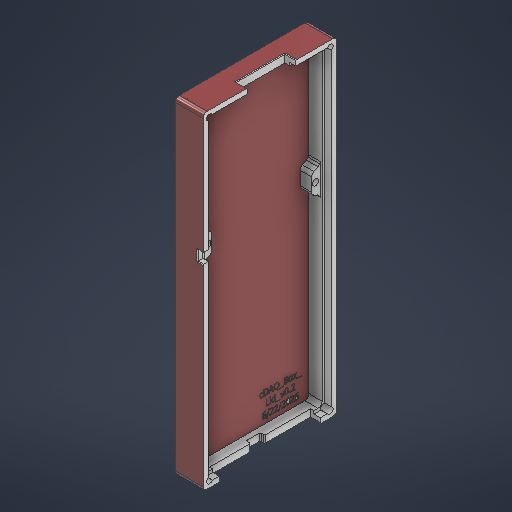
# Autodesk Inventor part: cDAQ_Box_Lid_v0.2
Saved by Autodesk Inventor 2027 (Build 310192000, 192)
## iProperties
Created: 2026-05-08
Part Number: cDAQ_Box_Lid_v0.2
Material: Generic
Document SubType Name: Modeling
Designer: giese
Density: 1 g/cm^3
Appearance: Default
Author: giese
Autodesk Inventor part; units mm, degrees
(part 1 of 2)
ref_plane "YZ Plane" through (0, 0, 0) normal (1, 0, 0) x (0, 1, 0)
ref_plane "XZ Plane" through (0, 0, 0) normal (0, 1, 0) x (-1, 0, 0)
ref_plane "XY Plane" through (0, 0, 0) normal (0, 0, 1) x (1, 0, 0)
sketch "Sketch1" plane through (0, 0, 0) normal (1, 0, 0) x (0, 1, 0)
  line L0 (50.7569, 48.4212) -> (-204.2591, 48.4212)
  line L1 (-204.2591, 48.4212) -> (-204.2591, -55.7188)
  line L2 (-204.2591, -55.7188) -> (50.7569, -55.7188)
  line L3 (50.7569, -55.7188) -> (50.7569, 48.4212)
  point P0 (0, 0)
  dimension "d0" = 104.14
  dimension "d1" = 255.016
  constraints: 8 end point, 2 parallel, 1 horizontal, 1 perpendicular
  measures "d0" distance of L2.end L0.start
  measures "d1" distance of L0.start L0.end
extrude "Extrusion1" add sketch "Sketch1" along normal blind 21.59
sketch "Sketch2" plane through (21.59, 0, 0) normal (1, 0, 0) x (0, 0, -1)
  line L0 (-42.0712, 44.4069) -> (49.3688, 44.4069)
  line L1 (49.3688, 44.4069) -> (49.3688, -197.9091)
  line L2 (49.3688, -197.9091) -> (-42.0712, -197.9091)
  line L3 (-42.0712, -197.9091) -> (-42.0712, 44.4069)
  line L4 (-48.4212, 50.7569) -> (-48.4212, -204.2591) projected
  line L5 (-48.4212, -204.2591) -> (55.7188, -204.2591) projected
  point P0 (0, 0)
  dimension "d4" = 91.44
  dimension "d5" = 242.316
  dimension "d6" = 6.35
  dimension "d7" = 6.35
  constraints: 8 end point, 2 parallel, 1 horizontal, 1 perpendicular
  measures "d4" distance of L0.start L0.end
  measures "d5" distance of L0.end L1.end
  measures "d6" distance between parallel lines of L4 L3
  measures "d7" distance between parallel lines of L5 L2
extrude "Extrusion2" cut sketch "Sketch2" against normal blind 15.24
sketch "Sketch3" plane through (0, 0, 0) normal (-1, 0, 0) x (0, 0, 1)
  circle A0 centre (-32.8588, 7.3229) radius 2
  line L0 (-55.7188, -204.2591) -> (-55.7188, 50.7569) projected
  line L1 (-55.7188, 50.7569) -> (48.4212, 50.7569) projected
  circle A1 centre (-14.36, 7.3229) radius 2
  circle A2 centre (4.1389, 7.3229) radius 2
  point P0 (0, 0)
  dimension "d10" = 22.86
  dimension "d11" = 43.434
  dimension "d12" = 43.434
  dimension "d13" = 18.4988
  dimension "d14" = 4
  dimension "d15" = 4
  dimension "d16" = 43.434
  dimension "d17" = 18.4988
  dimension "d18" = 36.9976
  dimension "d21" = 4
  constraints: 3 centre point
  measures "d10" distance from line of L0 A0.centre
  measures "d11" distance from line of L1 A0.centre
  measures "d12" distance from line of L1 A1.centre
  measures "d13" distance of A0.centre A1.centre
  measures "d14" diameter of A1
  measures "d15" diameter of A2
  measures "d16" distance from line of L1 A2.centre
  measures "d17" distance of A1.centre A2.centre
  measures "d18" distance of A0.centre A2.centre
  measures "d21" diameter of A0
extrude "Extrusion3" [suppressed]
sketch "Sketch6" plane through (0, 50.7569, 48.4212) normal (0, 1, 0) x (1, 0, 0)
  line L0 (21.59, 6.35) -> (21.59, 97.79) projected
  line L1 (12.954, 34.29) -> (21.59, 34.29)
  line L2 (21.59, 34.29) -> (21.59, 72.39)
  line L3 (21.59, 72.39) -> (12.954, 72.39)
  line L4 (12.954, 72.39) -> (12.954, 34.29)
  line L5 (0, 104.14) -> (21.59, 104.14) projected
  point P0 (0, 48.4212)
  point P1 (17.272, 72.39)
  point P2 (17.272, 34.29)
  dimension "d30" = 8.636
  dimension "d31" = 38.1
  dimension "d32" = 31.75
  constraints: 8 end point, 2 midpoint, 2 parallel, 1 horizontal, 1 perpendicular, 1 point on line
  measures "d30" distance between parallel lines of L0 L4
  measures "d31" distance of point (17.272, 72.39) point (17.272, 34.29)
  measures "d32" distance between parallel lines of L5 L3
extrude "Extrusion5" cut sketch "Sketch6" against normal blind 6.35
fillet "Fillet1" radius 3.175 4 edges at (10.795, 50.7569, -55.7188) (10.795, 50.7569, 48.4212) (10.795, -204.2591, 48.4212) (10.795, -204.2591, -55.7188)
sketch "Sketch7" plane through (21.59, 0, 0) normal (1, 0, 0) x (0, 0, -1)
  line L0 (-42.0712, -197.9091) -> (-42.0712, 44.4069) projected
  line L1 (-42.0712, 44.4069) -> (-42.3252, 44.4069)
  line L2 (-42.3252, 46.6929) -> (-44.2302, 46.6929)
  line L3 (-44.2302, 46.6929) -> (-44.2302, 51.0109)
  line L4 (-42.0712, -190.1621) -> (-42.0712, -197.9091)
  line L5 (49.3688, -197.9091) -> (-42.0712, -197.9091) projected
  line L6 (-40.4202, -200.1951) -> (-44.2302, -200.1951)
  line L7 (-44.2302, -200.1951) -> (-44.2302, -190.1621)
  line L8 (49.3688, 44.4069) -> (49.3688, -197.9091) projected
  line L9 (49.3688, -192.7021) -> (49.3688, -197.9091)
  line L10 (49.3688, -197.9091) -> (43.9078, -197.9091)
  line L11 (49.3688, -197.9091) -> (49.3688, -192.7021)
  line L12 (51.5278, -192.7021) -> (51.5278, -200.1951)
  line L13 (51.5278, -200.1951) -> (43.9078, -200.1951)
  line L14 (-42.0712, 44.4069) -> (49.3688, 44.4069) projected
  line L15 (42.0028, 44.4069) -> (49.3688, 44.4069)
  line L16 (51.5278, 48.4709) -> (51.5278, 46.6929)
  line L17 (51.5278, 46.6929) -> (42.0028, 46.6929)
  line L18 (-42.3252, 46.6929) -> (42.0028, 46.6929)
  line L19 (42.0028, 44.4069) -> (-42.3252, 44.4069)
  line L20 (51.5278, 48.4709) -> (51.5278, -192.7021)
  line L21 (44.2888, -195.2421) -> (44.2888, 44.4069)
  line L22 (43.9078, -197.9091) -> (-40.4202, -197.9091)
  line L23 (-40.4202, -200.1951) -> (43.9078, -200.1951)
  line L24 (-44.2302, -190.1621) -> (-44.2302, 51.0109)
  line L25 (-42.0712, 44.4069) -> (-42.0712, -190.1621)
  point P0 (0, 0)
  point P1 (-42.0712, 51.0109)
  point P2 (-44.2302, 48.9789)
  point P3 (49.3688, 48.4709)
  point P4 (51.5278, 46.6929)
  point P5 (-44.2302, 46.6929)
  point P6 (-42.0712, 50.7569)
  point P7 (46.8288, 50.7569)
  dimension "d34" = 2.286
  dimension "d35" = 2.159
  dimension "d38" = 2.159
  dimension "d39" = 2.286
  dimension "d42" = 2.286
  dimension "d43" = 2.159
  dimension "d46" = 2.286
  dimension "d47" = 2.159
  constraints: 44 end point, 7 point on line, 4 parallel, 4 perpendicular, 2 collinear, 2 horizontal, 2 vertical, 3 other
  measures "d34" distance between parallel lines of L2 L1
  measures "d35" distance between parallel lines of L0 L3
  measures "d38" distance between parallel lines of L7 L0
  measures "d39" distance between parallel lines of L5 L6
  measures "d42" distance between parallel lines of L5 L13
  measures "d46" distance between parallel lines of L14 L17
extrude "Extrusion6" cut sketch "Sketch7" against normal blind 5 contours L0 L14 L8 L5 | L18 L17 L20 L12 L13 L23 L6 L7 L24 L2
fillet "Fillet2" radius 3.175 8 edges at (19.09, 46.6929, 44.2302) (11.47, 44.4069, 42.0712) (19.09, 46.6929, -51.5278) (11.47, 44.4069, -49.3688) (11.47, -197.9091, 42.0712) (19.09, -200.1951, 44.2302) (11.47, -197.9091, -49.3688) (19.09, -200.1951, -51.5278)
sketch "Sketch11" plane through (16.59, 0, 0) normal (1, 0, 0) x (0, 0, -1)
  circle A0 centre (50.6388, 45.6769) radius 2.4005
  line L0 (52.5438, 50.7569) -> (23.9688, 50.7569) projected
  line L1 (55.7188, -201.0841) -> (55.7188, 47.5819) projected
  arc A1 (46.9238, 45.7719) -> (43.7488, 48.9469) centre (43.7488, 45.7719) ccw projected
  circle A2 centre (-43.3412, 45.6769) radius 2.4005
  line L2 (-48.4212, 47.5819) -> (-48.4212, -201.0841) projected
  line L3 (-14.1312, 50.7569) -> (-45.2462, 50.7569) projected
  circle A3 centre (50.6388, -199.1791) radius 2.4005
  line L4 (-45.2462, -204.2591) -> (52.5438, -204.2591) projected
  circle A4 centre (-43.3412, -199.1791) radius 2.4005
  circle A5 centre (45.5588, -45.7631) radius 2.4005
  circle A6 centre (-38.2612, -45.7631) radius 2.4005
  point P0 (0, 0)
  point P1 (45.9939, 48.017)
  point P2 (48.5528, -43.2993)
  point P3 (45.3778, -46.4743)
  point P4 (-30.4007, -42.8803)
  point P5 (-33.5757, -46.0553)
  point P6 (46.8288, 50.7569)
  point P7 (-42.0712, 50.7569)
  dimension "d58" = 4.801
  dimension "d59" = 5.08
  dimension "d60" = 5.08
  dimension "d61" = 4.801
  dimension "d62" = 4.801
  dimension "d63" = 5.08
  dimension "d64" = 5.08
  dimension "d65" = 4.801
  dimension "d66" = 5.08
  dimension "d67" = 5.08
  dimension "d76" = 5.08
  dimension "d77" = 5.08
  dimension "d114" = 4.801
  dimension "d115" = 96.52
  dimension "d116" = 10.16
  dimension "d117" = 4.801
  dimension "d118" = 96.52
  dimension "d119" = 10.16
  constraints: 6 centre point, 1 point on circle
  measures "d58" diameter of A0
  measures "d59" distance from line of L2 A2.centre
  measures "d60" distance from line of L3 A2.centre
  measures "d61" diameter of A2
  measures "d62" diameter of A3
  measures "d63" distance from line of L1 A3.centre
  measures "d64" distance from line of L4 A3.centre
  measures "d65" diameter of A4
  measures "d66" distance from line of L2 A4.centre
  measures "d67" distance from line of L4 A4.centre
  measures "d76" distance from line of L1 A0.centre
  measures "d77" distance from line of L0 A0.centre
  measures "d114" diameter of A5
  measures "d115" distance from line of A5.centre L0
  measures "d116" distance from line of L1 A5.centre
  measures "d117" diameter of A6
  measures "d118" distance from line of A6.centre L3
  measures "d119" distance from line of L2 A6.centre
extrude "Extrusion8" cut sketch "Sketch11" along normal blind 5.08 and the other way blind 17.78
sketch "Sketch13" plane through (6.35, 0, 0) normal (1, 0, 0) x (0, 0, -1)
  line L0 (14.7094, -174.4803) -> (39.7652, -174.4803) construction
  line L1 (39.7652, -174.4803) -> (39.7652, -183.3446) construction
  line L2 (39.7652, -183.3446) -> (14.7094, -183.3446) construction
  line L3 (14.7094, -183.3446) -> (14.7094, -174.4803) construction
  spline S0 degree 2 poles (12.7321, -179.2264) (12.3764, -179.2264) (11.7873, -179.0078) (11.5762, -178.7855) knots 0 0 0 1 2 2 2
  spline S1 degree 2 poles (11.5762, -178.7855) (11.365, -178.567) (11.1316, -177.8926) (11.1316, -177.4406) knots 0 0 0 1 2 2 2
  spline S2 degree 2 poles (11.1316, -177.4406) (11.1316, -176.9886) (11.3724, -176.3291) (11.5762, -176.1068) knots 0 0 0 1 2 2 2
  spline S3 degree 2 poles (11.5762, -176.1068) (11.7799, -175.8808) (12.3839, -175.64) (12.7321, -175.64) knots 0 0 0 1 2 2 2
  spline S4 degree 2 poles (12.7321, -175.64) (13.0137, -175.64) (13.5398, -175.7993) (13.7436, -175.903) knots 0 0 0 1 2 2 2
  line L4 (13.7436, -175.903) -> (13.7436, -176.5514)
  line L5 (13.7436, -176.5514) -> (13.7103, -176.5514)
  spline S5 degree 2 poles (13.7103, -176.5514) (13.6473, -176.4995) (13.4546, -176.3662) (13.3175, -176.2958) knots 0 0 0 1 2 2 2
  spline S6 degree 2 poles (13.3175, -176.2958) (13.1953, -176.2365) (12.8692, -176.1439) (12.721, -176.1439) knots 0 0 0 1 2 2 2
  spline S7 degree 2 poles (12.721, -176.1439) (12.2727, -176.1439) (11.7281, -176.8219) (11.7281, -177.4406) knots 0 0 0 1 2 2 2
  spline S8 degree 2 poles (11.7281, -177.4406) (11.7281, -178.0445) (12.2542, -178.7226) (12.721, -178.7226) knots 0 0 0 1 2 2 2
  spline S9 degree 2 poles (12.721, -178.7226) (13.0026, -178.7226) (13.5139, -178.4891) (13.7103, -178.3076) knots 0 0 0 1 2 2 2
  line L6 (13.7103, -178.3076) -> (13.7436, -178.3076)
  line L7 (13.7436, -178.3076) -> (13.7436, -178.956)
  spline S10 degree 2 poles (13.7436, -178.956) (13.6584, -178.9967) (13.399, -179.1116) (13.2953, -179.1375) knots 0 0 0 1 2 2 2
  spline S11 degree 2 poles (13.2953, -179.1375) (13.1471, -179.182) (12.9137, -179.2264) (12.7321, -179.2264) knots 0 0 0 1 2 2 2
  spline S12 degree 2 poles (17.9192, -176.8663) (17.9192, -177.4925) (17.4116, -178.5003) (16.9855, -178.7818) knots 0 0 0 1 2 2 2
  spline S13 degree 2 poles (16.9855, -178.7818) (16.6372, -179.0004) (15.9222, -179.1486) (15.3664, -179.1486) knots 0 0 0 1 2 2 2
  line L8 (15.3664, -179.1486) -> (14.3142, -179.1486)
  line L9 (14.3142, -179.1486) -> (14.3142, -174.5766)
  line L10 (14.3142, -174.5766) -> (15.3553, -174.5766)
  spline S14 degree 2 poles (15.3553, -174.5766) (16, -174.5766) (16.7336, -174.7693) (16.9929, -174.9397) knots 0 0 0 1 2 2 2
  spline S15 degree 2 poles (16.9929, -174.9397) (17.4338, -175.2324) (17.9192, -176.1994) (17.9192, -176.8663) knots 0 0 0 1 2 2 2
  spline S16 degree 2 poles (17.2856, -176.8589) (17.2856, -176.3328) (16.9373, -175.5881) (16.5928, -175.3769) knots 0 0 0 1 2 2 2
  spline S17 degree 2 poles (16.5928, -175.3769) (16.3482, -175.2324) (15.7962, -175.1028) (15.3849, -175.1028) knots 0 0 0 1 2 2 2
  line L11 (15.3849, -175.1028) -> (14.9218, -175.1028)
  line L12 (14.9218, -175.1028) -> (14.9218, -178.6225)
  line L13 (14.9218, -178.6225) -> (15.3849, -178.6225)
  spline S18 degree 2 poles (15.3849, -178.6225) (15.7888, -178.6225) (16.4001, -178.4929) (16.6483, -178.3187) knots 0 0 0 1 2 2 2
  spline S19 degree 2 poles (16.6483, -178.3187) (16.967, -178.1038) (17.2856, -177.3925) (17.2856, -176.8589) knots 0 0 0 1 2 2 2
  line L14 (18.0859, -179.1486) -> (19.6272, -174.5766)
  line L15 (19.6272, -174.5766) -> (20.3756, -174.5766)
  line L16 (20.3756, -174.5766) -> (21.9169, -179.1486)
  line L17 (21.9169, -179.1486) -> (21.2759, -179.1486)
  line L18 (21.2759, -179.1486) -> (20.8609, -177.8704)
  line L19 (20.8609, -177.8704) -> (19.1159, -177.8704)
  line L20 (19.1159, -177.8704) -> (18.7009, -179.1486)
  line L21 (18.7009, -179.1486) -> (18.0859, -179.1486)
  line L22 (20.6942, -177.3517) -> (19.9866, -175.1991)
  line L23 (19.9866, -175.1991) -> (19.2826, -177.3517)
  line L24 (19.2826, -177.3517) -> (20.6942, -177.3517)
  spline S20 degree 2 poles (26.148, -180.2676) (25.9813, -180.3083) (25.6182, -180.3528) (25.4367, -180.3528) knots 0 0 0 1 2 2 2
  spline S21 degree 2 poles (25.4367, -180.3528) (24.9217, -180.3528) (24.2807, -179.7785) (24.251, -179.245) knots 0 0 0 1 2 2 2
  spline S22 degree 2 poles (24.251, -179.245) (24.2103, -179.245) (24.1399, -179.245) (24.1103, -179.245) knots 0 0 0 1 2 2 2
  spline S23 degree 2 poles (24.1103, -179.245) (23.6471, -179.245) (22.9024, -178.93) (22.6357, -178.6225) knots 0 0 0 1 2 2 2
  spline S24 degree 2 poles (22.6357, -178.6225) (22.3726, -178.3187) (22.091, -177.4295) (22.091, -176.8663) knots 0 0 0 1 2 2 2
  spline S25 degree 2 poles (22.091, -176.8663) (22.091, -176.2884) (22.3763, -175.414) (22.6394, -175.1028) knots 0 0 0 1 2 2 2
  spline S26 degree 2 poles (22.6394, -175.1028) (22.9061, -174.7952) (23.6508, -174.4803) (24.1103, -174.4803) knots 0 0 0 1 2 2 2
  spline S27 degree 2 poles (24.1103, -174.4803) (24.5771, -174.4803) (25.3255, -174.8064) (25.5849, -175.1028) knots 0 0 0 1 2 2 2
  spline S28 degree 2 poles (25.5849, -175.1028) (25.8442, -175.4029) (26.1332, -176.2958) (26.1332, -176.8663) knots 0 0 0 1 2 2 2
  spline S29 degree 2 poles (26.1332, -176.8663) (26.1332, -177.7556) (25.4404, -178.9115) (24.8364, -179.1153) knots 0 0 0 1 2 2 2
  spline S30 degree 2 poles (24.8364, -179.1153) (24.8513, -179.2857) (24.9402, -179.5599) (25.0106, -179.6377) knots 0 0 0 1 2 2 2
  spline S31 degree 2 poles (25.0106, -179.6377) (25.0958, -179.734) (25.3292, -179.823) (25.5367, -179.823) knots 0 0 0 1 2 2 2
  spline S32 degree 2 poles (25.5367, -179.823) (25.659, -179.823) (25.9924, -179.7451) (26.0665, -179.7155) knots 0 0 0 1 2 2 2
  line L25 (26.0665, -179.7155) -> (26.148, -179.7155)
  line L26 (26.148, -179.7155) -> (26.148, -180.2676)
  spline S33 degree 2 poles (25.4996, -176.8663) (25.4996, -176.4106) (25.3033, -175.7104) (25.1254, -175.4807) knots 0 0 0 1 2 2 2
  spline S34 degree 2 poles (25.1254, -175.4807) (24.9439, -175.2435) (24.4326, -175.0064) (24.114, -175.0064) knots 0 0 0 1 2 2 2
  spline S35 degree 2 poles (24.114, -175.0064) (23.7842, -175.0064) (23.2877, -175.2361) (23.0988, -175.4807) knots 0 0 0 1 2 2 2
  spline S36 degree 2 poles (23.0988, -175.4807) (22.9172, -175.7141) (22.7246, -176.4217) (22.7246, -176.8663) knots 0 0 0 1 2 2 2
  spline S37 degree 2 poles (22.7246, -176.8663) (22.7246, -177.7667) (23.4804, -178.7263) (24.114, -178.7263) knots 0 0 0 1 2 2 2
  spline S38 degree 2 poles (24.114, -178.7263) (24.7475, -178.7263) (25.4996, -177.7667) (25.4996, -176.8663) knots 0 0 0 1 2 2 2
  line L27 (29.816, -180.0675) -> (26.2888, -180.0675)
  line L28 (26.2888, -180.0675) -> (26.2888, -179.671)
  line L29 (26.2888, -179.671) -> (29.816, -179.671)
  line L30 (29.816, -179.671) -> (29.816, -180.0675)
  spline S39 degree 2 poles (33.3321, -177.7444) (33.3321, -178.0853) (33.0727, -178.6077) (32.8578, -178.7781) knots 0 0 0 1 2 2 2
  spline S40 degree 2 poles (32.8578, -178.7781) (32.5985, -178.9782) (32.0094, -179.1486) (31.5425, -179.1486) knots 0 0 0 1 2 2 2
  line L31 (31.5425, -179.1486) -> (30.231, -179.1486)
  line L32 (30.231, -179.1486) -> (30.231, -174.5766)
  line L33 (30.231, -174.5766) -> (31.4425, -174.5766)
  spline S41 degree 2 poles (31.4425, -174.5766) (31.9316, -174.5766) (32.4206, -174.6396) (32.6429, -174.7619) knots 0 0 0 1 2 2 2
  spline S42 degree 2 poles (32.6429, -174.7619) (32.8912, -174.8916) (33.1172, -175.3176) (33.1172, -175.6066) knots 0 0 0 1 2 2 2
  spline S43 degree 2 poles (33.1172, -175.6066) (33.1172, -175.929) (32.7763, -176.4403) (32.4762, -176.5848) knots 0 0 0 1 2 2 2
  line L34 (32.4762, -176.5848) -> (32.4762, -176.607)
  spline S44 degree 2 poles (32.4762, -176.607) (32.8838, -176.7181) (33.3321, -177.3072) (33.3321, -177.7444) knots 0 0 0 1 2 2 2
  spline S45 degree 2 poles (32.6985, -177.7704) (32.6985, -177.511) (32.5503, -177.1776) (32.328, -177.059) knots 0 0 0 1 2 2 2
  spline S46 degree 2 poles (32.328, -177.059) (32.1835, -176.9849) (31.8426, -176.9404) (31.5277, -176.9404) knots 0 0 0 1 2 2 2
  line L35 (31.5277, -176.9404) -> (30.8386, -176.9404)
  line L36 (30.8386, -176.9404) -> (30.8386, -178.6299)
  line L37 (30.8386, -178.6299) -> (31.3313, -178.6299)
  spline S47 degree 2 poles (31.3313, -178.6299) (31.7315, -178.6299) (32.1909, -178.5558) (32.3688, -178.4373) knots 0 0 0 1 2 2 2
  spline S48 degree 2 poles (32.3688, -178.4373) (32.5392, -178.315) (32.6985, -178.0112) (32.6985, -177.7704) knots 0 0 0 1 2 2 2
  spline S49 degree 2 poles (32.4836, -175.6919) (32.4836, -175.5288) (32.3725, -175.2843) (32.2502, -175.2139) knots 0 0 0 1 2 2 2
  spline S50 degree 2 poles (32.2502, -175.2139) (32.102, -175.1324) (31.7426, -175.0953) (31.4203, -175.0953) knots 0 0 0 1 2 2 2
  line L38 (31.4203, -175.0953) -> (30.8386, -175.0953)
  line L39 (30.8386, -175.0953) -> (30.8386, -176.4329)
  line L40 (30.8386, -176.4329) -> (31.5277, -176.4329)
  spline S51 degree 2 poles (31.5277, -176.4329) (31.813, -176.4329) (32.0835, -176.3736) (32.228, -176.281) knots 0 0 0 1 2 2 2
  spline S52 degree 2 poles (32.228, -176.281) (32.3688, -176.192) (32.4836, -175.9067) (32.4836, -175.6919) knots 0 0 0 1 2 2 2
  spline S53 degree 2 poles (36.711, -177.4332) (36.711, -178.3002) (35.8774, -179.245) (35.1809, -179.245) knots 0 0 0 1 2 2 2
  spline S54 degree 2 poles (35.1809, -179.245) (34.4658, -179.245) (33.647, -178.2705) (33.647, -177.4332) knots 0 0 0 1 2 2 2
  spline S55 degree 2 poles (33.647, -177.4332) (33.647, -176.5736) (34.4917, -175.6215) (35.1809, -175.6215) knots 0 0 0 1 2 2 2
  spline S56 degree 2 poles (35.1809, -175.6215) (35.8774, -175.6215) (36.711, -176.5699) (36.711, -177.4332) knots 0 0 0 1 2 2 2
  spline S57 degree 2 poles (36.1145, -177.4332) (36.1145, -176.7663) (35.6292, -176.1179) (35.1809, -176.1179) knots 0 0 0 1 2 2 2
  spline S58 degree 2 poles (35.1809, -176.1179) (34.7326, -176.1179) (34.2435, -176.7663) (34.2435, -177.4332) knots 0 0 0 1 2 2 2
  spline S59 degree 2 poles (34.2435, -177.4332) (34.2435, -178.0816) (34.7326, -178.7485) (35.1809, -178.7485) knots 0 0 0 1 2 2 2
  spline S60 degree 2 poles (35.1809, -178.7485) (35.6255, -178.7485) (36.1145, -178.0927) (36.1145, -177.4332) knots 0 0 0 1 2 2 2
  line L41 (39.9678, -179.1486) -> (39.2601, -179.1486)
  line L42 (39.2601, -179.1486) -> (38.4265, -177.8593)
  line L43 (38.4265, -177.8593) -> (37.5706, -179.1486)
  line L44 (37.5706, -179.1486) -> (36.9148, -179.1486)
  line L45 (36.9148, -179.1486) -> (38.1041, -177.448)
  line L46 (38.1041, -177.448) -> (36.9259, -175.7178)
  line L47 (36.9259, -175.7178) -> (37.6336, -175.7178)
  line L48 (37.6336, -175.7178) -> (38.4635, -176.996)
  line L49 (38.4635, -176.996) -> (39.312, -175.7178)
  line L50 (39.312, -175.7178) -> (39.9678, -175.7178)
  line L51 (39.9678, -175.7178) -> (38.7859, -177.411)
  line L52 (38.7859, -177.411) -> (39.9678, -179.1486)
  line L53 (43.4764, -180.0675) -> (39.9492, -180.0675)
  line L54 (39.9492, -180.0675) -> (39.9492, -179.671)
  line L55 (39.9492, -179.671) -> (43.4764, -179.671)
  line L56 (43.4764, -179.671) -> (43.4764, -180.0675)
  line L57 (18.6657, -186.6763) -> (16.0166, -186.6763)
  line L58 (16.0166, -186.6763) -> (16.0166, -182.1043)
  line L59 (16.0166, -182.1043) -> (16.6243, -182.1043)
  line L60 (16.6243, -182.1043) -> (16.6243, -186.1354)
  line L61 (16.6243, -186.1354) -> (18.6657, -186.1354)
  line L62 (18.6657, -186.1354) -> (18.6657, -186.6763)
  line L63 (19.6883, -186.6763) -> (19.1103, -186.6763)
  line L64 (19.1103, -186.6763) -> (19.1103, -183.2455)
  line L65 (19.1103, -183.2455) -> (19.6883, -183.2455)
  line L66 (19.6883, -183.2455) -> (19.6883, -186.6763)
  line L67 (19.7291, -182.6749) -> (19.0733, -182.6749)
  line L68 (19.0733, -182.6749) -> (19.0733, -182.0747)
  line L69 (19.0733, -182.0747) -> (19.7291, -182.0747)
  line L70 (19.7291, -182.0747) -> (19.7291, -182.6749)
  line L71 (23.1747, -186.6763) -> (22.5968, -186.6763)
  line L72 (22.5968, -186.6763) -> (22.5968, -186.328)
  spline S61 degree 2 poles (22.5968, -186.328) (22.4634, -186.4392) (22.267, -186.5874) (22.1336, -186.6504) knots 0 0 0 1 2 2 2
  spline S62 degree 2 poles (22.1336, -186.6504) (22.0114, -186.7097) (21.7483, -186.7726) (21.5742, -186.7726) knots 0 0 0 1 2 2 2
  spline S63 degree 2 poles (21.5742, -186.7726) (21.2926, -186.7726) (20.8183, -186.5392) (20.6516, -186.3132) knots 0 0 0 1 2 2 2
  spline S64 degree 2 poles (20.6516, -186.3132) (20.4849, -186.0872) (20.2996, -185.4203) (20.2996, -184.9868) knots 0 0 0 1 2 2 2
  spline S65 degree 2 poles (20.2996, -184.9868) (20.2996, -184.5348) (20.5331, -183.8753) (20.7368, -183.6271) knots 0 0 0 1 2 2 2
  spline S66 degree 2 poles (20.7368, -183.6271) (20.9258, -183.4048) (21.4556, -183.1491) (21.7483, -183.1491) knots 0 0 0 1 2 2 2
  spline S67 degree 2 poles (21.7483, -183.1491) (22.004, -183.1491) (22.3856, -183.264) (22.5968, -183.3826) knots 0 0 0 1 2 2 2
  line L73 (22.5968, -183.3826) -> (22.5968, -181.9005)
  line L74 (22.5968, -181.9005) -> (23.1747, -181.9005)
  line L75 (23.1747, -181.9005) -> (23.1747, -186.6763)
  line L76 (22.5968, -185.8427) -> (22.5968, -183.8605)
  spline S68 degree 2 poles (22.5968, -183.8605) (22.3819, -183.7568) (22.041, -183.679) (21.8446, -183.679) knots 0 0 0 1 2 2 2
  spline S69 degree 2 poles (21.8446, -183.679) (21.4, -183.679) (20.8961, -184.3459) (20.8961, -184.9757) knots 0 0 0 1 2 2 2
  spline S70 degree 2 poles (20.8961, -184.9757) (20.8961, -185.5833) (21.2815, -186.2243) (21.7075, -186.2243) knots 0 0 0 1 2 2 2
  spline S71 degree 2 poles (21.7075, -186.2243) (21.9336, -186.2243) (22.393, -186.0168) (22.5968, -185.8427) knots 0 0 0 1 2 2 2
  line L77 (27.0724, -187.5952) -> (23.5452, -187.5952)
  line L78 (23.5452, -187.5952) -> (23.5452, -187.1987)
  line L79 (23.5452, -187.1987) -> (27.0724, -187.1987)
  line L80 (27.0724, -187.1987) -> (27.0724, -187.5952)
  line L81 (30.1365, -183.2455) -> (28.8434, -186.6763)
  line L82 (28.8434, -186.6763) -> (28.3247, -186.6763)
  line L83 (28.3247, -186.6763) -> (27.0428, -183.2455)
  line L84 (27.0428, -183.2455) -> (27.6689, -183.2455)
  line L85 (27.6689, -183.2455) -> (28.6063, -185.8871)
  line L86 (28.6063, -185.8871) -> (29.5363, -183.2455)
  line L87 (29.5363, -183.2455) -> (30.1365, -183.2455)
  spline S72 degree 2 poles (33.3339, -184.3903) (33.3339, -185.6204) (32.6188, -186.7726) (31.8741, -186.7726) knots 0 0 0 1 2 2 2
  spline S73 degree 2 poles (31.8741, -186.7726) (31.1183, -186.7726) (30.4107, -185.5982) (30.4107, -184.394) knots 0 0 0 1 2 2 2
  spline S74 degree 2 poles (30.4107, -184.394) (30.4107, -183.1565) (31.1257, -182.0117) (31.8741, -182.0117) knots 0 0 0 1 2 2 2
  spline S75 degree 2 poles (31.8741, -182.0117) (32.6263, -182.0117) (33.3339, -183.1973) (33.3339, -184.3903) knots 0 0 0 1 2 2 2
  spline S76 degree 2 poles (32.5484, -185.7834) (32.6374, -185.5574) (32.7115, -184.8609) (32.7115, -184.3903) knots 0 0 0 1 2 2 2
  spline S77 degree 2 poles (32.7115, -184.3903) (32.7115, -183.9198) (32.6374, -183.2269) (32.5447, -182.9935) knots 0 0 0 1 2 2 2
  spline S78 degree 2 poles (32.5447, -182.9935) (32.4521, -182.7601) (32.1298, -182.5193) (31.8741, -182.5193) knots 0 0 0 1 2 2 2
  spline S79 degree 2 poles (31.8741, -182.5193) (31.6185, -182.5193) (31.2887, -182.7601) (31.1924, -183.0009) knots 0 0 0 1 2 2 2
  spline S80 degree 2 poles (31.1924, -183.0009) (31.0998, -183.2344) (31.0331, -183.9457) (31.0331, -184.394) knots 0 0 0 1 2 2 2
  spline S81 degree 2 poles (31.0331, -184.394) (31.0331, -184.8757) (31.0924, -185.5204) (31.1887, -185.7723) knots 0 0 0 1 2 2 2
  spline S82 degree 2 poles (31.1887, -185.7723) (31.2776, -186.0094) (31.6074, -186.2651) (31.8741, -186.2651) knots 0 0 0 1 2 2 2
  spline S83 degree 2 poles (31.8741, -186.2651) (32.1261, -186.2651) (32.4558, -186.0242) (32.5484, -185.7834) knots 0 0 0 1 2 2 2
  line L88 (34.9011, -186.6763) -> (34.1675, -186.6763)
  line L89 (34.1675, -186.6763) -> (34.1675, -185.8019)
  line L90 (34.1675, -185.8019) -> (34.9011, -185.8019)
  line L91 (34.9011, -185.8019) -> (34.9011, -186.6763)
  line L92 (38.6432, -186.6763) -> (35.8237, -186.6763)
  line L93 (35.8237, -186.6763) -> (35.8237, -186.0279)
  spline S84 degree 2 poles (35.8237, -186.0279) (36.1275, -185.7427) (36.6684, -185.2128) (36.9278, -184.9275) knots 0 0 0 1 2 2 2
  spline S85 degree 2 poles (36.9278, -184.9275) (37.4502, -184.3533) (37.8318, -183.6641) (37.8318, -183.2973) knots 0 0 0 1 2 2 2
  spline S86 degree 2 poles (37.8318, -183.2973) (37.8318, -183.1047) (37.7133, -182.8157) (37.6058, -182.7231) knots 0 0 0 1 2 2 2
  spline S87 degree 2 poles (37.6058, -182.7231) (37.4984, -182.6304) (37.2168, -182.5378) (37.0463, -182.5378) knots 0 0 0 1 2 2 2
  spline S88 degree 2 poles (37.0463, -182.5378) (36.8833, -182.5378) (36.5499, -182.6193) (36.398, -182.6823) knots 0 0 0 1 2 2 2
  spline S89 degree 2 poles (36.398, -182.6823) (36.2683, -182.7342) (36.0275, -182.8824) (35.9534, -182.9342) knots 0 0 0 1 2 2 2
  line L94 (35.9534, -182.9342) -> (35.92, -182.9342)
  line L95 (35.92, -182.9342) -> (35.92, -182.2822)
  spline S90 degree 2 poles (35.92, -182.2822) (36.109, -182.1895) (36.787, -182.008) (37.0908, -182.008) knots 0 0 0 1 2 2 2
  spline S91 degree 2 poles (37.0908, -182.008) (37.7318, -182.008) (38.4543, -182.686) (38.4543, -183.264) knots 0 0 0 1 2 2 2
  spline S92 degree 2 poles (38.4543, -183.264) (38.4543, -183.5345) (38.3283, -183.9865) (38.2171, -184.1791) knots 0 0 0 1 2 2 2
  spline S93 degree 2 poles (38.2171, -184.1791) (38.106, -184.3792) (37.7836, -184.7719) (37.6058, -184.9609) knots 0 0 0 1 2 2 2
  spline S94 degree 2 poles (37.6058, -184.9609) (37.3168, -185.2758) (36.6092, -185.9501) (36.398, -186.1465) knots 0 0 0 1 2 2 2
  line L96 (36.398, -186.1465) -> (38.6432, -186.1465)
  line L97 (38.6432, -186.1465) -> (38.6432, -186.6763)
  spline S95 degree 2 poles (16.0481, -192.722) (16.0481, -193.074) (15.8147, -193.6705) (15.6183, -193.8705) knots 0 0 0 1 2 2 2
  spline S96 degree 2 poles (15.6183, -193.8705) (15.4146, -194.0817) (14.9033, -194.3003) (14.5958, -194.3003) knots 0 0 0 1 2 2 2
  spline S97 degree 2 poles (14.5958, -194.3003) (14.2882, -194.3003) (13.7806, -194.0928) (13.588, -193.8854) knots 0 0 0 1 2 2 2
  spline S98 degree 2 poles (13.588, -193.8854) (13.3509, -193.6371) (13.0841, -192.8035) (13.0841, -192.1959) knots 0 0 0 1 2 2 2
  spline S99 degree 2 poles (13.0841, -192.1959) (13.0841, -191.5994) (13.3286, -190.6398) (13.5843, -190.2841) knots 0 0 0 1 2 2 2
  spline S100 degree 2 poles (13.5843, -190.2841) (13.8325, -189.9358) (14.618, -189.5468) (15.133, -189.5468) knots 0 0 0 1 2 2 2
  spline S101 degree 2 poles (15.133, -189.5468) (15.2849, -189.5468) (15.5517, -189.5764) (15.6517, -189.6098) knots 0 0 0 1 2 2 2
  line L98 (15.6517, -189.6098) -> (15.6517, -190.1989)
  line L99 (15.6517, -190.1989) -> (15.6258, -190.1989)
  spline S102 degree 2 poles (15.6258, -190.1989) (15.5405, -190.1544) (15.2293, -190.0766) (15.0515, -190.0766) knots 0 0 0 1 2 2 2
  spline S103 degree 2 poles (15.0515, -190.0766) (14.4809, -190.0766) (13.7806, -190.8472) (13.714, -191.6031) knots 0 0 0 1 2 2 2
  spline S104 degree 2 poles (13.714, -191.6031) (13.9326, -191.4512) (14.392, -191.2844) (14.6661, -191.2844) knots 0 0 0 1 2 2 2
  spline S105 degree 2 poles (14.6661, -191.2844) (14.9329, -191.2844) (15.3331, -191.3919) (15.5517, -191.5549) knots 0 0 0 1 2 2 2
  spline S106 degree 2 poles (15.5517, -191.5549) (15.8036, -191.7439) (16.0481, -192.3293) (16.0481, -192.722) knots 0 0 0 1 2 2 2
  spline S107 degree 2 poles (15.4257, -192.7479) (15.4257, -192.4663) (15.2775, -192.0847) (15.1145, -191.9513) knots 0 0 0 1 2 2 2
  spline S108 degree 2 poles (15.1145, -191.9513) (14.9922, -191.855) (14.6884, -191.792) (14.5291, -191.792) knots 0 0 0 1 2 2 2
  spline S109 degree 2 poles (14.5291, -191.792) (14.3142, -191.792) (13.9103, -191.9217) (13.714, -192.044) knots 0 0 0 1 2 2 2
  spline S110 degree 2 poles (13.714, -192.044) (13.7103, -192.1107) (13.7028, -192.2366) (13.7028, -192.333) knots 0 0 0 1 2 2 2
  spline S111 degree 2 poles (13.7028, -192.333) (13.7028, -192.8072) (13.8881, -193.3889) (14.0289, -193.5408) knots 0 0 0 1 2 2 2
  spline S112 degree 2 poles (14.0289, -193.5408) (14.1586, -193.6853) (14.4401, -193.8001) (14.5995, -193.8001) knots 0 0 0 1 2 2 2
  spline S113 degree 2 poles (14.5995, -193.8001) (14.97, -193.8001) (15.4257, -193.274) (15.4257, -192.7479) knots 0 0 0 1 2 2 2
  line L100 (18.4897, -189.4282) -> (16.7002, -195.1969)
  line L101 (16.7002, -195.1969) -> (16.1815, -195.1969)
  line L102 (16.1815, -195.1969) -> (17.9636, -189.4282)
  line L103 (17.9636, -189.4282) -> (18.4897, -189.4282)
  line L104 (21.8131, -194.204) -> (18.9936, -194.204)
  line L105 (18.9936, -194.204) -> (18.9936, -193.5556)
  spline S114 degree 2 poles (18.9936, -193.5556) (19.2974, -193.2703) (19.8384, -192.7405) (20.0977, -192.4552) knots 0 0 0 1 2 2 2
  spline S115 degree 2 poles (20.0977, -192.4552) (20.6201, -191.8809) (21.0017, -191.1918) (21.0017, -190.825) knots 0 0 0 1 2 2 2
  spline S116 degree 2 poles (21.0017, -190.825) (21.0017, -190.6324) (20.8832, -190.3434) (20.7757, -190.2507) knots 0 0 0 1 2 2 2
  spline S117 degree 2 poles (20.7757, -190.2507) (20.6683, -190.1581) (20.3867, -190.0655) (20.2163, -190.0655) knots 0 0 0 1 2 2 2
  spline S118 degree 2 poles (20.2163, -190.0655) (20.0533, -190.0655) (19.7198, -190.147) (19.5679, -190.21) knots 0 0 0 1 2 2 2
  spline S119 degree 2 poles (19.5679, -190.21) (19.4382, -190.2618) (19.1974, -190.4101) (19.1233, -190.4619) knots 0 0 0 1 2 2 2
  line L106 (19.1233, -190.4619) -> (19.0899, -190.4619)
  line L107 (19.0899, -190.4619) -> (19.0899, -189.8098)
  spline S120 degree 2 poles (19.0899, -189.8098) (19.2789, -189.7172) (19.9569, -189.5357) (20.2607, -189.5357) knots 0 0 0 1 2 2 2
  spline S121 degree 2 poles (20.2607, -189.5357) (20.9017, -189.5357) (21.6242, -190.2137) (21.6242, -190.7917) knots 0 0 0 1 2 2 2
  spline S122 degree 2 poles (21.6242, -190.7917) (21.6242, -191.0621) (21.4982, -191.5141) (21.3871, -191.7068) knots 0 0 0 1 2 2 2
  spline S123 degree 2 poles (21.3871, -191.7068) (21.2759, -191.9069) (20.9536, -192.2996) (20.7757, -192.4886) knots 0 0 0 1 2 2 2
  spline S124 degree 2 poles (20.7757, -192.4886) (20.4867, -192.8035) (19.7791, -193.4778) (19.5679, -193.6742) knots 0 0 0 1 2 2 2
  line L108 (19.5679, -193.6742) -> (21.8131, -193.6742)
  line L109 (21.8131, -193.6742) -> (21.8131, -194.204)
  line L110 (25.244, -194.204) -> (22.4245, -194.204)
  line L111 (22.4245, -194.204) -> (22.4245, -193.5556)
  spline S125 degree 2 poles (22.4245, -193.5556) (22.7283, -193.2703) (23.2692, -192.7405) (23.5286, -192.4552) knots 0 0 0 1 2 2 2
  spline S126 degree 2 poles (23.5286, -192.4552) (24.051, -191.8809) (24.4326, -191.1918) (24.4326, -190.825) knots 0 0 0 1 2 2 2
  spline S127 degree 2 poles (24.4326, -190.825) (24.4326, -190.6324) (24.314, -190.3434) (24.2066, -190.2507) knots 0 0 0 1 2 2 2
  spline S128 degree 2 poles (24.2066, -190.2507) (24.0991, -190.1581) (23.8176, -190.0655) (23.6471, -190.0655) knots 0 0 0 1 2 2 2
  spline S129 degree 2 poles (23.6471, -190.0655) (23.4841, -190.0655) (23.1507, -190.147) (22.9987, -190.21) knots 0 0 0 1 2 2 2
  spline S130 degree 2 poles (22.9987, -190.21) (22.8691, -190.2618) (22.6282, -190.4101) (22.5541, -190.4619) knots 0 0 0 1 2 2 2
  line L112 (22.5541, -190.4619) -> (22.5208, -190.4619)
  line L113 (22.5208, -190.4619) -> (22.5208, -189.8098)
  spline S131 degree 2 poles (22.5208, -189.8098) (22.7098, -189.7172) (23.3878, -189.5357) (23.6916, -189.5357) knots 0 0 0 1 2 2 2
  spline S132 degree 2 poles (23.6916, -189.5357) (24.3326, -189.5357) (25.055, -190.2137) (25.055, -190.7917) knots 0 0 0 1 2 2 2
  spline S133 degree 2 poles (25.055, -190.7917) (25.055, -191.0621) (24.9291, -191.5141) (24.8179, -191.7068) knots 0 0 0 1 2 2 2
  spline S134 degree 2 poles (24.8179, -191.7068) (24.7068, -191.9069) (24.3844, -192.2996) (24.2066, -192.4886) knots 0 0 0 1 2 2 2
  spline S135 degree 2 poles (24.2066, -192.4886) (23.9176, -192.8035) (23.2099, -193.4778) (22.9987, -193.6742) knots 0 0 0 1 2 2 2
  line L114 (22.9987, -193.6742) -> (25.244, -193.6742)
  line L115 (25.244, -193.6742) -> (25.244, -194.204)
  line L116 (27.756, -189.4282) -> (25.9665, -195.1969)
  line L117 (25.9665, -195.1969) -> (25.4478, -195.1969)
  line L118 (25.4478, -195.1969) -> (27.2299, -189.4282)
  line L119 (27.2299, -189.4282) -> (27.756, -189.4282)
  line L120 (31.0794, -194.204) -> (28.2599, -194.204)
  line L121 (28.2599, -194.204) -> (28.2599, -193.5556)
  spline S136 degree 2 poles (28.2599, -193.5556) (28.5637, -193.2703) (29.1046, -192.7405) (29.364, -192.4552) knots 0 0 0 1 2 2 2
  spline S137 degree 2 poles (29.364, -192.4552) (29.8864, -191.8809) (30.268, -191.1918) (30.268, -190.825) knots 0 0 0 1 2 2 2
  spline S138 degree 2 poles (30.268, -190.825) (30.268, -190.6324) (30.1494, -190.3434) (30.042, -190.2507) knots 0 0 0 1 2 2 2
  spline S139 degree 2 poles (30.042, -190.2507) (29.9346, -190.1581) (29.653, -190.0655) (29.4825, -190.0655) knots 0 0 0 1 2 2 2
  spline S140 degree 2 poles (29.4825, -190.0655) (29.3195, -190.0655) (28.9861, -190.147) (28.8342, -190.21) knots 0 0 0 1 2 2 2
  spline S141 degree 2 poles (28.8342, -190.21) (28.7045, -190.2618) (28.4637, -190.4101) (28.3896, -190.4619) knots 0 0 0 1 2 2 2
  line L122 (28.3896, -190.4619) -> (28.3562, -190.4619)
  line L123 (28.3562, -190.4619) -> (28.3562, -189.8098)
  spline S142 degree 2 poles (28.3562, -189.8098) (28.5452, -189.7172) (29.2232, -189.5357) (29.527, -189.5357) knots 0 0 0 1 2 2 2
  spline S143 degree 2 poles (29.527, -189.5357) (30.168, -189.5357) (30.8905, -190.2137) (30.8905, -190.7917) knots 0 0 0 1 2 2 2
  spline S144 degree 2 poles (30.8905, -190.7917) (30.8905, -191.0621) (30.7645, -191.5141) (30.6533, -191.7068) knots 0 0 0 1 2 2 2
  spline S145 degree 2 poles (30.6533, -191.7068) (30.5422, -191.9069) (30.2198, -192.2996) (30.042, -192.4886) knots 0 0 0 1 2 2 2
  spline S146 degree 2 poles (30.042, -192.4886) (29.753, -192.8035) (29.0453, -193.4778) (28.8342, -193.6742) knots 0 0 0 1 2 2 2
  line L124 (28.8342, -193.6742) -> (31.0794, -193.6742)
  line L125 (31.0794, -193.6742) -> (31.0794, -194.204)
  spline S147 degree 2 poles (34.5362, -191.918) (34.5362, -193.1481) (33.8211, -194.3003) (33.0764, -194.3003) knots 0 0 0 1 2 2 2
  spline S148 degree 2 poles (33.0764, -194.3003) (32.3206, -194.3003) (31.6129, -193.1258) (31.6129, -191.9217) knots 0 0 0 1 2 2 2
  spline S149 degree 2 poles (31.6129, -191.9217) (31.6129, -190.6842) (32.328, -189.5394) (33.0764, -189.5394) knots 0 0 0 1 2 2 2
  spline S150 degree 2 poles (33.0764, -189.5394) (33.8285, -189.5394) (34.5362, -190.725) (34.5362, -191.918) knots 0 0 0 1 2 2 2
  spline S151 degree 2 poles (33.7507, -193.3111) (33.8396, -193.0851) (33.9138, -192.3885) (33.9138, -191.918) knots 0 0 0 1 2 2 2
  spline S152 degree 2 poles (33.9138, -191.918) (33.9138, -191.4475) (33.8396, -190.7546) (33.747, -190.5212) knots 0 0 0 1 2 2 2
  spline S153 degree 2 poles (33.747, -190.5212) (33.6544, -190.2878) (33.3321, -190.047) (33.0764, -190.047) knots 0 0 0 1 2 2 2
  spline S154 degree 2 poles (33.0764, -190.047) (32.8208, -190.047) (32.491, -190.2878) (32.3947, -190.5286) knots 0 0 0 1 2 2 2
  spline S155 degree 2 poles (32.3947, -190.5286) (32.3021, -190.762) (32.2354, -191.4734) (32.2354, -191.9217) knots 0 0 0 1 2 2 2
  spline S156 degree 2 poles (32.2354, -191.9217) (32.2354, -192.4034) (32.2947, -193.048) (32.391, -193.3) knots 0 0 0 1 2 2 2
  spline S157 degree 2 poles (32.391, -193.3) (32.4799, -193.5371) (32.8097, -193.7927) (33.0764, -193.7927) knots 0 0 0 1 2 2 2
  spline S158 degree 2 poles (33.0764, -193.7927) (33.3284, -193.7927) (33.6581, -193.5519) (33.7507, -193.3111) knots 0 0 0 1 2 2 2
  line L126 (37.9411, -194.204) -> (35.1216, -194.204)
  line L127 (35.1216, -194.204) -> (35.1216, -193.5556)
  spline S159 degree 2 poles (35.1216, -193.5556) (35.4254, -193.2703) (35.9663, -192.7405) (36.2257, -192.4552) knots 0 0 0 1 2 2 2
  spline S160 degree 2 poles (36.2257, -192.4552) (36.7481, -191.8809) (37.1297, -191.1918) (37.1297, -190.825) knots 0 0 0 1 2 2 2
  spline S161 degree 2 poles (37.1297, -190.825) (37.1297, -190.6324) (37.0112, -190.3434) (36.9037, -190.2507) knots 0 0 0 1 2 2 2
  spline S162 degree 2 poles (36.9037, -190.2507) (36.7963, -190.1581) (36.5147, -190.0655) (36.3442, -190.0655) knots 0 0 0 1 2 2 2
  spline S163 degree 2 poles (36.3442, -190.0655) (36.1812, -190.0655) (35.8478, -190.147) (35.6959, -190.21) knots 0 0 0 1 2 2 2
  spline S164 degree 2 poles (35.6959, -190.21) (35.5662, -190.2618) (35.3254, -190.4101) (35.2513, -190.4619) knots 0 0 0 1 2 2 2
  line L128 (35.2513, -190.4619) -> (35.2179, -190.4619)
  line L129 (35.2179, -190.4619) -> (35.2179, -189.8098)
  spline S165 degree 2 poles (35.2179, -189.8098) (35.4069, -189.7172) (36.0849, -189.5357) (36.3887, -189.5357) knots 0 0 0 1 2 2 2
  spline S166 degree 2 poles (36.3887, -189.5357) (37.0297, -189.5357) (37.7522, -190.2137) (37.7522, -190.7917) knots 0 0 0 1 2 2 2
  spline S167 degree 2 poles (37.7522, -190.7917) (37.7522, -191.0621) (37.6262, -191.5141) (37.515, -191.7068) knots 0 0 0 1 2 2 2
  spline S168 degree 2 poles (37.515, -191.7068) (37.4039, -191.9069) (37.0815, -192.2996) (36.9037, -192.4886) knots 0 0 0 1 2 2 2
  spline S169 degree 2 poles (36.9037, -192.4886) (36.6147, -192.8035) (35.9071, -193.4778) (35.6959, -193.6742) knots 0 0 0 1 2 2 2
  line L130 (35.6959, -193.6742) -> (37.9411, -193.6742)
  line L131 (37.9411, -193.6742) -> (37.9411, -194.204)
  spline S170 degree 2 poles (41.4424, -192.722) (41.4424, -193.074) (41.2089, -193.6705) (41.0126, -193.8705) knots 0 0 0 1 2 2 2
  spline S171 degree 2 poles (41.0126, -193.8705) (40.8088, -194.0817) (40.2975, -194.3003) (39.99, -194.3003) knots 0 0 0 1 2 2 2
  spline S172 degree 2 poles (39.99, -194.3003) (39.6825, -194.3003) (39.1749, -194.0928) (38.9822, -193.8854) knots 0 0 0 1 2 2 2
  spline S173 degree 2 poles (38.9822, -193.8854) (38.7451, -193.6371) (38.4783, -192.8035) (38.4783, -192.1959) knots 0 0 0 1 2 2 2
  spline S174 degree 2 poles (38.4783, -192.1959) (38.4783, -191.5994) (38.7229, -190.6398) (38.9785, -190.2841) knots 0 0 0 1 2 2 2
  spline S175 degree 2 poles (38.9785, -190.2841) (39.2268, -189.9358) (40.0122, -189.5468) (40.5272, -189.5468) knots 0 0 0 1 2 2 2
  spline S176 degree 2 poles (40.5272, -189.5468) (40.6791, -189.5468) (40.9459, -189.5764) (41.0459, -189.6098) knots 0 0 0 1 2 2 2
  line L132 (41.0459, -189.6098) -> (41.0459, -190.1989)
  line L133 (41.0459, -190.1989) -> (41.02, -190.1989)
  spline S177 degree 2 poles (41.02, -190.1989) (40.9348, -190.1544) (40.6235, -190.0766) (40.4457, -190.0766) knots 0 0 0 1 2 2 2
  spline S178 degree 2 poles (40.4457, -190.0766) (39.8751, -190.0766) (39.1749, -190.8472) (39.1082, -191.6031) knots 0 0 0 1 2 2 2
  spline S179 degree 2 poles (39.1082, -191.6031) (39.3268, -191.4512) (39.7862, -191.2844) (40.0604, -191.2844) knots 0 0 0 1 2 2 2
  spline S180 degree 2 poles (40.0604, -191.2844) (40.3271, -191.2844) (40.7273, -191.3919) (40.9459, -191.5549) knots 0 0 0 1 2 2 2
  spline S181 degree 2 poles (40.9459, -191.5549) (41.1978, -191.7439) (41.4424, -192.3293) (41.4424, -192.722) knots 0 0 0 1 2 2 2
  spline S182 degree 2 poles (40.8199, -192.7479) (40.8199, -192.4663) (40.6717, -192.0847) (40.5087, -191.9513) knots 0 0 0 1 2 2 2
  spline S183 degree 2 poles (40.5087, -191.9513) (40.3864, -191.855) (40.0826, -191.792) (39.9233, -191.792) knots 0 0 0 1 2 2 2
  spline S184 degree 2 poles (39.9233, -191.792) (39.7084, -191.792) (39.3046, -191.9217) (39.1082, -192.044) knots 0 0 0 1 2 2 2
  spline S185 degree 2 poles (39.1082, -192.044) (39.1045, -192.1107) (39.0971, -192.2366) (39.0971, -192.333) knots 0 0 0 1 2 2 2
  spline S186 degree 2 poles (39.0971, -192.333) (39.0971, -192.8072) (39.2823, -193.3889) (39.4231, -193.5408) knots 0 0 0 1 2 2 2
  spline S187 degree 2 poles (39.4231, -193.5408) (39.5528, -193.6853) (39.8344, -193.8001) (39.9937, -193.8001) knots 0 0 0 1 2 2 2
  spline S188 degree 2 poles (39.9937, -193.8001) (40.3642, -193.8001) (40.8199, -193.274) (40.8199, -192.7479) knots 0 0 0 1 2 2 2
  point P0 (0, 0)
  constraints: 2 other
emboss "Emboss1" sketch "Sketch13" operation cut depth 2.54 direction (-1, 0, 0)